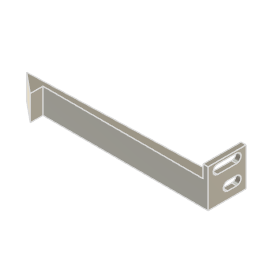
Babyproofing latch (Autodesk Fusion 360 design; units mm, degrees)
Autodesk Fusion 360 part; units mm, degrees
sketch "Sketch1" plane through (0, 0, 0) normal (0, 0, 1) x (1, 0, 0)
  line L0 (0, 0) -> (-65, 0)
  line L1 (-65, 0) -> (-65, -5)
  line L2 (-65, -5) -> (-73, 1.6)
  line L3 (-73, 1.6) -> (-2, 4)
  line L4 (-2, 4) -> (-2, 15)
  line L5 (-2, 15) -> (0, 15)
  line L6 (0, 15) -> (0, 0)
  line L7 (-2, 4) -> (-2, 0)
  dimension "d1" = 65
  dimension "d2" = 15
  dimension "d3" = 2
  dimension "d4" = 5
  dimension "d5" = 8
  dimension "d6" = 1.6
  dimension "d7" = 4
  constraint coincident L0.start L6.end
  constraint horizontal L0
  constraint perpendicular L0 L1
  constraint perpendicular L0 L4
  constraint perpendicular L4 L5
  constraint perpendicular L5 L6
  constraint coincident L0 L7.end
  constraint perpendicular L0 L7
  measures "d1" distance of L0.start L1
  measures "d2" distance of L0.start L5.end
  measures "d3" distance of L4.end L5.end
  measures "d4" distance of L0.end L1.end
  measures "d5" horizontal distance of L0.end L2.end
  measures "d6" vertical distance of L0.end L2.end
  measures "d7" vertical distance of L0.start L3.end
extrude "Extrude1" add sketch "Sketch1" along normal blind 15 contours L0 L4 L5 L6 L7
extrude "Extrude2" add sketch "Sketch1" along normal blind 10 contours L0 L1 L2 L3 L7
sketch "Sketch2" plane through (0, 0, 0) normal (1, 0, 0) x (0, 1, 0)
  line L0 (0, 0) -> (15, 0)
  line L1 (15, 0) -> (15, 15)
  line L2 (15, 15) -> (0, 15)
  line L3 (0, 15) -> (0, 0)
  line L4 (4, 10) -> (0, 10) construction
  line L5 (4, 0) -> (4, 10) construction
  line L6 (3.75, 10.5322) -> (11.25, 10.5322)
  arc A0 (11.25, 10.5322) -> (11.25, 14.0322) centre (11.25, 12.2822) ccw
  line L7 (11.25, 14.0322) -> (3.75, 14.0322)
  arc A1 (3.75, 14.0322) -> (3.75, 10.5322) centre (3.75, 12.2822) ccw
  line L8 (3.75, 12.2822) -> (11.25, 12.2822) construction
  line L9 (7.5, 15) -> (7.5, 0) construction
  line L10 (7.75, 2.9241) -> (11.25, 2.9241)
  arc A2 (11.25, 2.9241) -> (11.25, 6.4241) centre (11.25, 4.6741) ccw
  line L11 (11.25, 6.4241) -> (7.75, 6.4241)
  arc A3 (7.75, 6.4241) -> (7.75, 2.9241) centre (7.75, 4.6741) ccw
  line L12 (6, 4.6741) -> (13, 4.6741) construction
  dimension "d12" = 3.5
  dimension "d13" = 3.5
  dimension "d14" = 2
  dimension "d15" = 2
  dimension "d16" = 2
  dimension "d17" = 2
  constraint tangent L6 A0
  constraint tangent A0 L7
  constraint parallel L6 L7
  constraint tangent L7 A1
  constraint tangent L6 A1
  constraint horizontal L8
  constraint midpoint L2 L9.start
  constraint midpoint L0 L9.end
  constraint tangent L10 A2
  constraint tangent A2 L11
  constraint parallel L10 L11
  constraint tangent L11 A3
  constraint tangent L10 A3
  constraint midpoint A3 L12.start
  constraint midpoint A2 L12.end
  constraint horizontal L12
  measures "d12" distance of L6 L7
  measures "d13" distance of L10 L11
  measures "d14" distance of L1 A0
  measures "d15" distance of L1 L12.end
  measures "d16" distance of L5 A3
  measures "d17" distance of L3 A1
extrude "Extrude3" cut sketch "Sketch2" against normal up to surface (2 mm away) contours L6 A0 L7 A1 | L10 A2 L11 A3
fillet "Fillet1" radius 1 1 edges at (-2, 4, 5)
equation "d13 = d12"
named bodies: "Babyproofing Latch"
